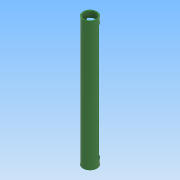
# Autodesk Inventor part: Pancake_Tilt Pipe
Saved by Autodesk Inventor 2018.1 (Build 221171000, 171)
## iProperties
Created: 2019-02-25
Part Number: Pancake_Tilt Pipe
Material: PVC-Piping
Document SubType Name: Modeling
Designer: James
Density: 1.4 g/cm^3
Appearance: Smooth - Dark Forest Green
Author: James
Autodesk Inventor part; units mm, degrees
ref_plane "YZ Plane" through (0, 0, 0) normal (1, 0, 0) x (0, 1, 0)
ref_plane "XZ Plane" through (0, 0, 0) normal (0, 1, 0) x (-1, 0, 0)
ref_plane "XY Plane" through (0, 0, 0) normal (0, 0, 1) x (1, 0, 0)
sketch "Sketch1" plane through (0, 0, 0) normal (0, 0, 1) x (1, 0, 0)
  circle A0 centre (0, 0) radius 20
  circle A1 centre (0, 0) radius 23
  dimension "d0" = 40
  dimension "d1" = 46
  constraints: 2 centre point, 2 coincident
  measures "d0" diameter of A0
  measures "d1" diameter of A1
extrude "Extrusion1" add sketch "Sketch1" along normal mid plane 425
sketch "Sketch2" plane through (0, 0, 0) normal (1, 0, 0) x (0, 1, 0)
  line L0 (0, 280) -> (0, -280) projected
  line L1 (-280, 0) -> (280, 0) projected
  point P0 (0, 0)
  point P1 (0, 150)
  point P2 (0, 0)
  point P3 (0, -150)
  dimension "d4" = 150
  dimension "d5" = 150
  constraints: 2 midpoint, 2 vertical alignment
  measures "d4" distance of point (0, 0) point (0, 150)
  measures "d5" distance of point (0, -150) point (0, 0)
hole "Hole1" at (0, 0, 150) at (0, 0, 0) at (0, 0, -150) direction (-1, 0, 0) diameter 4.5 end through all clearance for "Flat Head Machine Screw" size "M4" standard "Ansi Metric M Profile"
sketch "Sketch3" plane through (0, 0, 0) normal (1, 0, 0) x (0, 1, 0)
  line L0 (23, -192.5) -> (7, -192.5)
  line L1 (7, -192.5) -> (7, 192.5)
  line L2 (7, 192.5) -> (23, 192.5)
  line L3 (23, 192.5) -> (23, -192.5)
  line L4 (23, 212.5) -> (-23, 212.5) projected
  line L5 (-23, -212.5) -> (23, -212.5) projected
  line L6 (0, 364) -> (0, -364) projected
  point P0 (0, 0)
  dimension "d13" = 20
  dimension "d14" = 20
  dimension "d15" = 7
  constraints: 8 end point, 2 parallel, 1 horizontal, 1 perpendicular, 1 vertical alignment
  measures "d13" distance between parallel lines of L4 L2
  measures "d14" distance between parallel lines of L5 L0
  measures "d15" distance between parallel lines of L6 L1
extrude "Extrusion2" cut sketch "Sketch3" along normal through all both and the other way through all
fillet "Fillet1" radius 2 4 edges at (20.3219, 7, -192.5) (-20.3219, 7, -192.5) (20.3219, 7, 192.5) (-20.3219, 7, 192.5)
equation "\"d5\" = d4"
body "Solid1"
